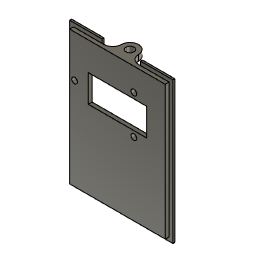
SolderingStation_DisplayBackplate (Autodesk Fusion 360 design; units mm, degrees)
Autodesk Fusion 360 part; units mm, degrees
sketch "Sketch2" plane through (0, 0, 0) normal (0, 1, 0) x (1, 0, 0)
  line L0 (24.9, -34.9) -> (-24.9, -34.9)
  line L1 (-24.9, -34.9) -> (-24.9, 34.9)
  line L2 (-24.9, 34.9) -> (24.9, 34.9)
  line L3 (24.9, 34.9) -> (24.9, -34.9)
  line L4 (24.9, -34.9) -> (-24.9, 34.9) construction
  line L5 (-24.9, -34.9) -> (24.9, 34.9) construction
  dimension "d1" = 49.8
  dimension "d2" = 69.8
  constraint horizontal L0
  constraint perpendicular L0 L1
  constraint parallel L0 L2
  constraint parallel L1 L3
  constraint coincident L4 origin
  constraint coincident L5 origin
  measures "d1" distance of L1.end L2.end
  measures "d2" distance of L0.end L1.end
extrude "Extrude1" add sketch "Sketch2" along normal blind 2
sketch "Sketch3" plane through (0, 0, 0) normal (0, -1, 0) x (1, 0, 0)
  line L0 (-24.9, -34.9) -> (24.9, -34.9)
  line L1 (24.9, -34.9) -> (24.9, 34.9)
  line L2 (24.9, 34.9) -> (-24.9, 34.9)
  line L3 (-24.9, 34.9) -> (-24.9, -34.9)
  line L4 (15.2, 20.15) -> (-15.2, 20.15)
  line L5 (-15.2, 20.15) -> (-15.2, 5.85)
  line L6 (-15.2, 5.85) -> (15.2, 5.85)
  line L7 (15.2, 5.85) -> (15.2, 20.15)
  line L8 (15.2, 20.15) -> (-15.2, 5.85) construction
  line L9 (-15.2, 20.15) -> (15.2, 5.85) construction
  line L10 (17.85, 23.03) -> (-22.3, 23.03) construction
  line L11 (-22.3, 23.03) -> (-22.3, 2.97) construction
  line L12 (-22.3, 2.97) -> (17.85, 2.97) construction
  line L13 (17.85, 2.97) -> (17.85, 23.03) construction
  line L14 (17.85, 23.03) -> (-22.3, 2.97) construction
  line L15 (-22.3, 23.03) -> (17.85, 2.97) construction
  line L16 (0, 13) -> (15.2, 13) construction
  circle A0 centre (8.55, 23.03) radius 1.5
  circle A1 centre (8.55, 2.97) radius 1.5
  circle A2 centre (-22.3, 13) radius 1.5
  point P0 (0, 13)
  point P1 (-2.225, 13)
  dimension "d5" = 30.4
  dimension "d6" = 14.3
  dimension "d7" = 40.15
  dimension "d8" = 20.06
  dimension "d10" = 2.65
  dimension "d11" = 3
  dimension "d12" = 9.3
  dimension "d13" = 3
  constraint horizontal L4
  constraint perpendicular L4 L5
  constraint parallel L4 L6
  constraint parallel L5 L7
  constraint coincident L8 P0
  constraint coincident L9 P0
  constraint horizontal L10
  constraint perpendicular L10 L11
  constraint parallel L10 L12
  constraint parallel L11 L13
  constraint coincident L14 P1
  constraint coincident L15 P1
  constraint coincident P0 L16.start
  constraint midpoint L7 L16.end
  constraint coincident L10 A0.centre
  constraint symmetric L16 A0 A1
  constraint midpoint L11 A2.centre
  measures "d5" distance of L5.end L6.end
  measures "d6" distance of L4.end L5.end
  measures "d7" distance of L11.end L12.end
  measures "d8" distance of L10.end L11.end
  measures "d10" distance of L7 L13
  measures "d11" diameter of A0
  measures "d12" distance of L13 A0.centre
  measures "d13" diameter of A2
extrude "Extrude2" cut sketch "Sketch3" against normal blind 2 contours L4 L5 L6 L7 | A0 | A1 | A2
sketch "Sketch5" plane through (0, 2, 0) normal (0, 1, 0) x (-1, 0, 0)
  circle A0 centre (22.3, 13) radius 1.5
  circle A1 centre (-8.55, 2.97) radius 1.5
  line L0 (-15.2, 20.15) -> (15.2, 20.15)
  line L1 (15.2, 20.15) -> (15.2, 5.85)
  line L2 (15.2, 5.85) -> (-15.2, 5.85)
  line L3 (-15.2, 5.85) -> (-15.2, 20.15)
  circle A2 centre (-8.55, 23.03) radius 1.5
  line L4 (-24.9, -34.9) -> (24.9, -34.9)
  line L5 (24.9, -34.9) -> (24.9, 34.9)
  line L6 (24.9, 34.9) -> (-24.9, 34.9)
  line L7 (-24.9, 34.9) -> (-24.9, -34.9)
  line L8 (-26.9, -36.9) -> (26.9, -36.9)
  line L9 (26.9, -36.9) -> (26.9, 36.9)
  line L10 (26.9, 36.9) -> (-26.9, 36.9)
  line L11 (-26.9, 36.9) -> (-26.9, -36.9)
  line L12 (-23.9, 33.9) -> (-23.9, -33.9)
  line L13 (-23.9, -33.9) -> (23.9, -33.9)
  line L14 (23.9, -33.9) -> (23.9, 33.9)
  line L15 (23.9, 33.9) -> (-23.9, 33.9)
  line L16 (0, 34.9) -> (0, -34.9) construction
  line L17 (-24.9, 0) -> (24.9, 0) construction
  line L18 (-10, 33.9) -> (10, 33.9)
  line L19 (10, 33.9) -> (10, 36.9)
  line L20 (10, 36.9) -> (-10, 36.9)
  line L21 (-10, 36.9) -> (-10, 33.9)
  line L22 (10, -36.9) -> (-10, -36.9)
  line L23 (10, -33.9) -> (10, -36.9)
  line L24 (-10, -36.9) -> (-10, -33.9)
  line L25 (-10, -33.9) -> (10, -33.9)
  dimension "d17" = 2
  dimension "d18" = -1
  dimension "d34" = 20
  dimension "d35" = 10
  constraint midpoint L6 L16.start
  constraint midpoint L4 L16.end
  constraint midpoint L7 L17.start
  constraint midpoint L5 L17.end
  constraint horizontal L18
  constraint vertical L19
  constraint horizontal L20
  constraint vertical L21
  constraint coincident L10 L19.end
  constraint coincident L15 L18.start
  constraint symmetric L17 L18.start L24.end
  constraint symmetric L17 L18.end L23.start
  constraint symmetric L17 L19.end L22.start
  constraint symmetric L17 L20.end L22.end
  measures "d34" distance of L19.end L20.end
  measures "d35" distance of L16 L21
extrude "Extrude3" add sketch "Sketch5" along normal blind 1 contours L4 L6 L7 L12 L13 L15 L21 L24 | L4 L6 L7 L8 L10 L11 L21 L24 | L4 L5 L6 L13 L14 L15 L19 L23 | L4 L5 L6 L8 L9 L10 L19 L23
sketch "Sketch6" plane through (0, 2, 0) normal (0, 1, 0) x (-1, 0, 0)
  line L0 (-23.9, 33.9) -> (-23.9, -33.9)
  line L1 (-23.9, -33.9) -> (-10, -33.9)
  line L2 (23.9, -33.9) -> (23.9, 33.9)
  line L3 (-10, 33.9) -> (-23.9, 33.9)
  circle A0 centre (22.3, 13) radius 1.5
  circle A1 centre (-8.55, 2.97) radius 1.5
  line L4 (-15.2, 20.15) -> (15.2, 20.15)
  line L5 (15.2, 20.15) -> (15.2, 5.85)
  line L6 (15.2, 5.85) -> (-15.2, 5.85)
  line L7 (-15.2, 5.85) -> (-15.2, 20.15)
  circle A2 centre (-8.55, 23.03) radius 1.5
  circle A3 centre (22.3, 13) radius 3
  line L8 (10, 33.9) -> (10, 34.9)
  line L9 (10, 34.9) -> (-10, 34.9)
  line L10 (-10, 34.9) -> (-10, 33.9)
  line L11 (-10, -33.9) -> (-10, -34.9)
  line L12 (-10, -34.9) -> (10, -34.9)
  line L13 (10, -34.9) -> (10, -33.9)
  line L14 (10, -33.9) -> (23.9, -33.9)
  line L15 (23.9, 33.9) -> (10, 33.9)
  dimension "d21" = 6
  constraint concentric A0 A3
  measures "d21" diameter of A3
extrude "Extrude4" cut sketch "Sketch6" along normal blind 1 contours L2 A3 | L2 A3
sketch "Sketch9" plane through (0, 2, 0) normal (0, 1, 0) x (-1, 0, 0)
  circle A0 centre (22.3, 13) radius 1.5
  line L0 (23.9, 15.5377) -> (23.9, 33.9)
  line L1 (23.9, 33.9) -> (10, 33.9)
  line L2 (10, 33.9) -> (10, 34.9)
  line L3 (10, 34.9) -> (-10, 34.9)
  line L4 (-10, 34.9) -> (-10, 33.9)
  line L5 (-10, 33.9) -> (-23.9, 33.9)
  line L6 (-23.9, 33.9) -> (-23.9, -33.9)
  line L7 (-23.9, -33.9) -> (-10, -33.9)
  line L8 (-10, -33.9) -> (-10, -34.9)
  line L9 (-10, -34.9) -> (10, -34.9)
  line L10 (10, -34.9) -> (10, -33.9)
  line L11 (10, -33.9) -> (23.9, -33.9)
  line L12 (23.9, -33.9) -> (23.9, 10.4623)
  arc A1 (23.9, 10.4623) -> (24.9, 11.5033) centre (22.3, 13) ccw
  line L13 (24.9, 11.5033) -> (24.9, 14.4967)
  arc A2 (24.9, 14.4967) -> (23.9, 15.5377) centre (22.3, 13) ccw
  circle A3 centre (-8.55, 23.03) radius 1.5
  line L14 (-15.2, 20.15) -> (15.2, 20.15)
  line L15 (15.2, 20.15) -> (15.2, 5.85)
  line L16 (15.2, 5.85) -> (-15.2, 5.85)
  line L17 (-15.2, 5.85) -> (-15.2, 20.15)
  circle A4 centre (-8.55, 2.97) radius 1.5
  line L18 (0, 34.9) -> (0, -34.9) construction
  line L19 (-27, 0) -> (27, 0) construction
  line L20 (-4.5, 34.9) -> (4.5, 34.9)
  line L21 (4.5, 34.9) -> (4.5, 31.9)
  line L22 (4.5, 31.9) -> (-4.5, 31.9)
  line L23 (-4.5, 31.9) -> (-4.5, 34.9)
  line L24 (-4.5, -34.9) -> (4.5, -34.9)
  line L25 (-4.5, -31.9) -> (-4.5, -34.9)
  line L26 (4.5, -31.9) -> (-4.5, -31.9)
  line L27 (4.5, -34.9) -> (4.5, -31.9)
  dimension "d36" = 9
  dimension "d37" = 3
  dimension "d38" = 4.5
  constraint midpoint L3 L18.start
  constraint midpoint L9 L18.end
  constraint perpendicular L12 L19
  constraint horizontal L20
  constraint vertical L21
  constraint horizontal L22
  constraint vertical L23
  constraint coincident L3 L20.start
  constraint symmetric L19 L20.start L24.start
  constraint symmetric L19 L20.end L24.end
  constraint symmetric L19 L21.end L26.start
  constraint symmetric L19 L22.end L25.start
  measures "d36" distance of L20.start L20.end
  measures "d37" distance of L20.start L22.end
  measures "d38" distance of L18 L21
extrude "Extrude7" add sketch "Sketch9" along normal blind 9 contours L3 L20 L21 L22 L23 | L9 L24 L25 L26 L27
sketch "Sketch10" plane through (0, 0, -34.9) normal (0, 0, -1) x (1, 0, 0)
  line L0 (24.9, 0) -> (-24.9, 0)
  line L1 (-24.9, 0) -> (-24.9, -2)
  line L2 (-24.9, -2) -> (-10, -2)
  line L3 (-10, -2) -> (-4.5, -2)
  line L4 (-4.5, -2) -> (-4.5, -11)
  line L5 (-4.5, -11) -> (4.5, -11)
  line L6 (4.5, -11) -> (4.5, -2)
  line L7 (4.5, -2) -> (10, -2)
  line L8 (10, -2) -> (24.9, -2)
  line L9 (24.9, -2) -> (24.9, 0)
  line L10 (-4.5, -2) -> (4.5, -11) construction
  line L11 (4.5, -2) -> (-4.5, -11) construction
  circle A0 centre (0, -6.5) radius 2.15
  dimension "d41" = 4.3
  constraint coincident L3.end L4.start
  constraint coincident L5.end L6.start
  constraint coincident L6.end L7.start
  constraint coincident L4.end L5.start
  constraint midpoint L11 A0.centre
  measures "d41" diameter of A0
extrude "Extrude8" cut sketch "Sketch10" against normal blind 72 contours A0
fillet "Fillet2" radius 4.5 8 edges at (4.5, 2, 33.4) (4.5, 11, 33.4) (-4.5, 11, 33.4) (-4.5, 2, 33.4) (-4.5, 11, -33.4) (-4.5, 2, -33.4) (4.5, 2, -33.4) (4.5, 11, -33.4)
